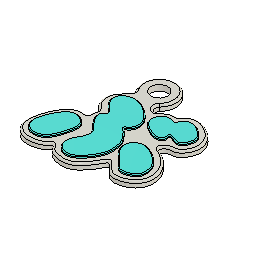
Azusa Keychain v20 (Autodesk Fusion 360 design; units mm, degrees)
Autodesk Fusion 360 part; units mm, degrees
sketch "bu body v1" plane through (0, 0, 0) normal (0, 0, 1) x (1, 0, 0)
  spline S0 degree 5 poles (6, 10.5) (6.0651, 10.4849) (6.1928, 10.4539) (6.3776, 10.4055) (6.613, 10.3384) (6.8974, 10.2472) (7.1797, 10.1429) (7.466, 10.0202) (7.7577, 9.8771) (8.05, 9.7182) (8.3341, 9.552) (8.6001, 9.3883) (8.8398, 9.2348) (9.05, 9.0947) (9.235, 8.9629) (9.4055, 8.8281) (9.573, 8.6777) (9.747, 8.5011) (9.9302, 8.2941) (10.1197, 8.0582) (10.3096, 7.798) (10.4927, 7.52) (10.6625, 7.2306) (10.8153, 6.9344) (10.9497, 6.6341) (11.0654, 6.3312) (11.1624, 6.0254) (11.2404, 5.7155) (11.2976, 5.3993) (11.3305, 5.0737) (11.3355, 4.7363) (11.3087, 4.3852) (11.2474, 4.0202) (11.1503, 3.6436) (11.0188, 3.2605) (10.8558, 2.8783) (10.6654, 2.5057) (10.4525, 2.1523) (10.2219, 1.8273) (9.9778, 1.5389) (9.7234, 1.2938) (9.4603, 1.0961) (9.1896, 0.9468) (8.9122, 0.8434) (8.6294, 0.7793) (8.3433, 0.743) (8.0573, 0.7185) (7.776, 0.6885) (7.5048, 0.638) (7.25, 0.557) (7.0183, 0.4446) (6.8165, 0.3081) (6.6486, 0.1589) (6.515, 0.0091) (6.4091, -0.1323) (6.3217, -0.2616) (6.2485, -0.3814) (6.1987, -0.5028) (6.1902, -0.6388) (6.2341, -0.7899) (6.3285, -0.9399) (6.4663, -1.0704) (6.6417, -1.1757) (6.8525, -1.2658) (7.0972, -1.3573) (7.3745, -1.4687) (7.6812, -1.612) (8.0118, -1.7924) (8.3596, -2.0101) (8.7171, -2.2614) (9.0767, -2.5407) (9.4313, -2.8418) (9.775, -3.1594) (10.1032, -3.4905) (10.413, -3.8338) (10.7021, -4.1895) (10.9689, -4.5584) (11.2124, -4.942) (11.4312, -5.3415) (11.624, -5.7579) (11.7883, -6.1909) (11.9216, -6.6394) (12.0205, -7.1012) (12.0818, -7.5733) (12.1022, -8.0519) (12.0791, -8.5327) (12.0101, -9.0107) (11.8939, -9.4807) (11.7303, -9.9369) (11.5201, -10.3736) (11.265, -10.7854) (10.9681, -11.1673) (10.6331, -11.5151) (10.265, -11.8256) (9.8696, -12.0971) (9.4537, -12.3293) (9.025, -12.5239) (8.5913, -12.6831) (8.1601, -12.8097) (7.7382, -12.9059) (7.331, -12.9733) (6.9418, -13.0114) (6.5716, -13.0176) (6.2187, -12.9866) (5.8795, -12.9125) (5.5505, -12.7901) (5.2287, -12.6178) (4.9132, -12.3982) (4.6064, -12.1412) (4.3142, -11.8637) (4.0441, -11.5857) (3.803, -11.3264) (3.595, -11.1004) (3.4204, -10.9147) (3.2725, -10.7632) (3.1384, -10.6297) (3.0052, -10.5012) (2.8642, -10.3791) (2.716, -10.2915) (2.5657, -10.2748) (2.4174, -10.3536) (2.2703, -10.5251) (2.1212, -10.7708) (1.9652, -11.0642) (1.7985, -11.3816) (1.6192, -11.7081) (1.427, -12.0355) (1.2221, -12.3604) (1.0058, -12.6828) (0.779, -13.0038) (0.5424, -13.3247) (0.2959, -13.6445) (0.0388, -13.9607) (-0.2302, -14.2697) (-0.5126, -14.5671) (-0.81, -14.848) (-1.1239, -15.1074) (-1.4556, -15.3407) (-1.8061, -15.5438) (-2.1756, -15.7134) (-2.5639, -15.8468) (-2.97, -15.9427) (-3.3917, -16.0007) (-3.8261, -16.0215) (-4.2689, -16.0076) (-4.7147, -15.9624) (-5.1574, -15.89) (-5.5901, -15.7943) (-6.0055, -15.6791) (-6.3959, -15.5471) (-6.7538, -15.3998) (-7.0715, -15.2363) (-7.3427, -15.0549) (-7.5644, -14.8549) (-7.7387, -14.638) (-7.8741, -14.41) (-7.9888, -14.1834) (-8.107, -13.9758) (-8.2489, -13.8056) (-8.4241, -13.6881) (-8.6195, -13.6311) (-8.8065, -13.6345) (-8.9599, -13.6934) (-9.078, -13.8005) (-9.1852, -13.9476) (-9.3132, -14.1249) (-9.485, -14.3213) (-9.7075, -14.5243) (-9.9776, -14.7218) (-10.2854, -14.9032) (-10.618, -15.0604) (-10.9635, -15.19) (-11.3136, -15.2929) (-11.6626, -15.3727) (-12.0072, -15.4345) (-12.3459, -15.4832) (-12.6791, -15.5221) (-13.008, -15.5512) (-13.3348, -15.5671) (-13.6619, -15.5645) (-13.9911, -15.5373) (-14.3239, -15.4801) (-14.6601, -15.389) (-14.9979, -15.2631) (-15.3341, -15.1035) (-15.6647, -14.9127) (-15.9847, -14.6934) (-16.2891, -14.4483) (-16.573, -14.179) (-16.8318, -13.8856) (-17.0613, -13.5667) (-17.2583, -13.2206) (-17.4199, -12.8452) (-17.544, -12.4388) (-17.6295, -12.0005) (-17.6761, -11.531) (-17.6844, -11.0324) (-17.6557, -10.508) (-17.5918, -9.9623) (-17.495, -9.4004) (-17.3677, -8.8281) (-17.2123, -8.2516) (-17.0313, -7.6772) (-16.8268, -7.1111) (-16.6005, -6.5593) (-16.3537, -6.0273) (-16.0876, -5.5203) (-15.8033, -5.0428) (-15.5022, -4.599) (-15.186, -4.1925) (-14.8569, -3.8264) (-14.5177, -3.503) (-14.1722, -3.2241) (-13.8251, -2.9907) (-13.4819, -2.8028) (-13.148, -2.6597) (-12.8282, -2.5589) (-12.5269, -2.4967) (-12.2466, -2.4675) (-11.9883, -2.4639) (-11.7515, -2.4769) (-11.5355, -2.4971) (-11.3399, -2.5147) (-11.1659, -2.5205) (-11.014, -2.508) (-10.8814, -2.4756) (-10.7587, -2.4294) (-10.6395, -2.3746) (-10.5367, -2.2995) (-10.4776, -2.1794) (-10.4711, -2.0027) (-10.4932, -1.7833) (-10.5096, -1.5453) (-10.4911, -1.3123) (-10.4352, -1.0926) (-10.3601, -0.8833) (-10.2924, -0.6772) (-10.2568, -0.4686) (-10.2659, -0.2603) (-10.3233, -0.0582) (-10.4256, 0.132) (-10.5661, 0.3095) (-10.7356, 0.4791) (-10.9244, 0.6487) (-11.1235, 0.8281) (-11.3257, 1.0264) (-11.5261, 1.2515) (-11.7209, 1.5098) (-11.9059, 1.8056) (-12.0764, 2.1406) (-12.2256, 2.5137) (-12.3447, 2.9206) (-12.4243, 3.3548) (-12.456, 3.8077) (-12.4336, 4.2692) (-12.3541, 4.7284) (-12.2194, 5.1739) (-12.0375, 5.5944) (-11.8227, 5.979) (-11.5921, 6.3193) (-11.3628, 6.6094) (-11.15, 6.8481) (-10.9635, 7.0391) (-10.8053, 7.1928) (-10.6677, 7.3267) (-10.5389, 7.4579) (-10.4069, 7.5986) (-10.2651, 7.7477) (-10.1137, 7.8962) (-9.9597, 8.0362) (-9.857, 8.18) (-9.8, 8.3) (-9.745, 8.49) (-9.7278, 8.731) (-9.7317, 8.9564) (-9.8441, 9.2185) (-9.9813, 9.4744) (-10.1241, 9.7107) (-10.2447, 9.9217) (-10.3356, 10.0776) (-10.3927, 10.1973) (-10.4249, 10.2758) (-10.4373, 10.3081) knots 0 0 0 0 0 0 0.00286533 0.00573066 0.00859599 0.01146132 0.01432665 0.01719198 0.02005731 0.02292264 0.02578797 0.0286533 0.03151862 0.03438395 0.03724928 0.04011461 0.04297994 0.04584527 0.0487106 0.05157593 0.05444126 0.05730659 0.06017192 0.06303725 0.06590258 0.06876791 0.07163324 0.07449857 0.0773639 0.08022923 0.08309456 0.08595989 0.08882521 0.09169054 0.09455587 0.0974212 0.10028653 0.10315186 0.10601719 0.10888252 0.11174785 0.11461318 0.11747851 0.12034384 0.12320917 0.1260745 0.12893983 0.13180516 0.13467049 0.13753582 0.14040115 0.14326648 0.14613181 0.14899713 0.15186246 0.15472779 0.15759312 0.16045845 0.16332378 0.16618911 0.16905444 0.17191977 0.1747851 0.17765043 0.18051576 0.18338109 0.18624642 0.18911175 0.19197708 0.19484241 0.19770774 0.20057307 0.2034384 0.20630372 0.20916905 0.21203438 0.21489971 0.21776504 0.22063037 0.2234957 0.22636103 0.22922636 0.23209169 0.23495702 0.23782235 0.24068768 0.24355301 0.24641834 0.24928367 0.252149 0.25501433 0.25787966 0.26074499 0.26361032 0.26647564 0.26934097 0.2722063 0.27507163 0.27793696 0.28080229 0.28366762 0.28653295 0.28939828 0.29226361 0.29512894 0.29799427 0.3008596 0.30372493 0.30659026 0.30945559 0.31232092 0.31518625 0.31805158 0.32091691 0.32378223 0.32664756 0.32951289 0.33237822 0.33524355 0.33810888 0.34097421 0.34383954 0.34670487 0.3495702 0.35243553 0.35530086 0.35816619 0.36103152 0.36389685 0.36676218 0.36962751 0.37249284 0.37535817 0.3782235 0.38108883 0.38395415 0.38681948 0.38968481 0.39255014 0.39541547 0.3982808 0.40114613 0.40401146 0.40687679 0.40974212 0.41260745 0.41547278 0.41833811 0.42120344 0.42406877 0.4269341 0.42979943 0.43266476 0.43553009 0.43839542 0.44126074 0.44412607 0.4469914 0.44985673 0.45272206 0.45558739 0.45845272 0.46131805 0.46418338 0.46704871 0.46991404 0.47277937 0.4756447 0.47851003 0.48137536 0.48424069 0.48710602 0.48997135 0.49283668 0.49570201 0.49856734 0.50143266 0.50429799 0.50716332 0.51002865 0.51289398 0.51575931 0.51862464 0.52148997 0.5243553 0.52722063 0.53008596 0.53295129 0.53581662 0.53868195 0.54154728 0.54441261 0.54727794 0.55014327 0.5530086 0.55587393 0.55873926 0.56160458 0.56446991 0.56733524 0.57020057 0.5730659 0.57593123 0.57879656 0.58166189 0.58452722 0.58739255 0.59025788 0.59312321 0.59598854 0.59885387 0.6017192 0.60458453 0.60744986 0.61031519 0.61318052 0.61604585 0.61891117 0.6217765 0.62464183 0.62750716 0.63037249 0.63323782 0.63610315 0.63896848 0.64183381 0.64469914 0.64756447 0.6504298 0.65329513 0.65616046 0.65902579 0.66189112 0.66475645 0.66762178 0.67048711 0.67335244 0.67621777 0.67908309 0.68194842 0.68481375 0.68767908 0.69054441 0.69340974 0.69627507 0.6991404 0.70200573 0.70487106 0.70773639 0.71060172 0.71346705 0.71633238 0.71919771 0.72206304 0.72492837 0.7277937 0.73065903 0.73352436 0.73638968 0.73925501 0.74212034 0.74498567 0.747851 0.75071633 0.75358166 0.75644699 0.75931232 0.76217765 0.76504298 0.76790831 0.77077364 0.77363897 0.7765043 0.77936963 0.78223496 0.78510029 0.78796562 0.79083095 0.79369628 0.79563186 0.79563186 0.79563186 0.79563186 0.79563186 0.79563186
  spline S1 degree 5 poles (-3.3703, 9.0276) (-3.381, 9.0158) (-3.4138, 8.9797) (-3.4691, 8.9165) (-3.5512, 8.8116) (-3.65, 8.65) (-3.6951, 8.4217) (-3.7207, 8.1798) (-3.6788, 7.9044) (-3.5655, 7.6182) (-3.3861, 7.3491) (-3.1557, 7.123) (-2.8982, 6.9575) (-2.6471, 6.8539) (-2.436, 6.8022) (-2.285, 6.7911) (-2.1899, 6.8154) (-2.1093, 6.8846) (-1.9979, 7.0086) (-1.8382, 7.1828) (-1.6328, 7.393) (-1.3945, 7.6201) (-1.1381, 7.8446) (-0.8694, 8.0524) (-0.5856, 8.2353) (-0.2811, 8.3893) (0.0484, 8.5132) (0.401, 8.6078) (0.7641, 8.6744) (1.1095, 8.7132) (1.4051, 8.7268) (1.626, 8.7231) (1.765, 8.7176) (1.8465, 8.7381) (1.9263, 8.8217) (2.0517, 8.9877) (2.2451, 9.2284) (2.5124, 9.5201) (2.8461, 9.8284) (3.2304, 10.1171) (3.6459, 10.3546) (4.0742, 10.5226) (4.5004, 10.6184) (4.9132, 10.6491) (5.3042, 10.6288) (5.5959, 10.5852) (5.8024, 10.5444) (5.9349, 10.5151) (6, 10.5) knots 0.875389 0.875389 0.875389 0.875389 0.875389 0.875389 0.876791 0.879656 0.882521 0.885387 0.888252 0.891117 0.893983 0.896848 0.899713 0.902579 0.905444 0.908309 0.911175 0.91404 0.916905 0.919771 0.922636 0.925501 0.928367 0.931232 0.934097 0.936963 0.939828 0.942693 0.945559 0.948424 0.951289 0.954155 0.95702 0.959885 0.962751 0.965616 0.968481 0.971347 0.974212 0.977077 0.979943 0.982808 0.985673 0.988539 0.991404 0.994269 0.997135 1 1 1 1 1 1
  arc A0 (-3.3703, 9.0276) -> (-10.2449, 9.9216) centre (-6.474, 12.0397) ccw
  circle A1 centre (-6.474, 12.0397) radius 2.1568
  point P0 (-10.4373, 10.3081)
  constraint coincident P0 A0
  constraint coincident S0 A0.end
  constraint concentric A0 A1
extrude "Extrude1" add sketch "bu body v1" along normal blind 1.5 contours S0 S1 A0
fillet "Fillet1" radius 0.5 3 edges at (-5.9163, 16.3285, 1.5) (-2.5581, -15.8345, 1.5) (-0.5045, 8.2701, 1.5)
sketch "bu middle v1" plane through (0, 0, 1.5) normal (0, 0, 1) x (1, 0, 0)
  spline S0 degree 5 poles (-1.4999, -2.0615) (-1.4521, -2.1021) (-1.322, -2.2306) (-1.044, -2.5481) (-0.6778, -2.9696) (-0.2817, -3.4492) (0.0829, -3.9373) (0.3768, -4.3995) (0.5894, -4.8223) (0.7286, -5.2064) (0.8143, -5.563) (0.8704, -5.9091) (0.9184, -6.2631) (0.9683, -6.6396) (1.017, -7.048) (1.0539, -7.4934) (1.0632, -7.9766) (1.0285, -8.4949) (0.9356, -9.0427) (0.7771, -9.6116) (0.5538, -10.1915) (0.2725, -10.7708) (-0.0555, -11.3373) (-0.4164, -11.879) (-0.7956, -12.3849) (-1.1794, -12.8453) (-1.5568, -13.2529) (-1.9215, -13.6035) (-2.273, -13.8964) (-2.6146, -14.1332) (-2.952, -14.3172) (-3.2914, -14.4522) (-3.6375, -14.5415) (-3.992, -14.587) (-4.3524, -14.5885) (-4.7141, -14.5456) (-5.0707, -14.4578) (-5.4157, -14.3258) (-5.7436, -14.1527) (-6.0503, -13.9438) (-6.3321, -13.7053) (-6.5857, -13.4427) (-6.8075, -13.1599) (-6.9927, -12.8578) (-7.1356, -12.5336) (-7.2314, -12.1851) (-7.2771, -11.8123) (-7.2732, -11.4202) (-7.2252, -11.0224) (-7.1435, -10.6398) (-7.04, -10.2937) (-6.9262, -9.9999) (-6.8104, -9.7632) (-6.6944, -9.5691) (-6.5746, -9.3869) (-6.4458, -9.1836) (-6.3055, -8.9353) (-6.1572, -8.6393) (-6.0094, -8.3067) (-5.8732, -7.9558) (-5.7618, -7.6061) (-5.6881, -7.2702) (-5.6638, -6.9502) (-5.6978, -6.6424) (-5.7949, -6.3396) (-5.9548, -6.0356) (-6.1697, -5.7279) (-6.4271, -5.4179) (-6.7114, -5.1081) (-7.007, -4.801) (-7.3, -4.4976) (-7.5813, -4.195) (-7.8475, -3.8862) (-8.0975, -3.5632) (-8.3304, -3.219) (-8.5425, -2.85) (-8.7254, -2.4587) (-8.8624, -2.0562) (-8.9319, -1.6607) (-8.9158, -1.2916) (-8.8068, -0.9655) (-8.6146, -0.6915) (-8.376, -0.4656) (-8.1494, -0.2713) (-7.996, -0.0868) (-7.9661, 0.111) (-8.08, 0.3395) (-8.3267, 0.6091) (-8.6751, 0.9243) (-9.0816, 1.2843) (-9.4994, 1.684) (-9.8869, 2.1143) (-10.2166, 2.5631) (-10.4728, 3.0167) (-10.6496, 3.4611) (-10.7483, 3.8836) (-10.7755, 4.274) (-10.7405, 4.6257) (-10.6533, 4.9382) (-10.5229, 5.2158) (-10.3572, 5.4651) (-10.162, 5.6936) (-9.9406, 5.9064) (-9.6933, 6.1054) (-9.4187, 6.2899) (-9.1145, 6.4564) (-8.7787, 6.5999) (-8.4102, 6.714) (-8.0096, 6.7914) (-7.5789, 6.8251) (-7.1209, 6.809) (-6.6398, 6.7387) (-6.1406, 6.6123) (-5.629, 6.4313) (-5.1118, 6.2001) (-4.5957, 5.9249) (-4.0883, 5.6133) (-3.5968, 5.2733) (-3.1288, 4.9124) (-2.6912, 4.5374) (-2.2908, 4.1529) (-1.9336, 3.7615) (-1.625, 3.3642) (-1.369, 2.9618) (-1.1685, 2.5555) (-1.0248, 2.1482) (-0.9375, 1.7447) (-0.9041, 1.3538) (-0.92, 0.986) (-0.9783, 0.6514) (-1.0696, 0.3562) (-1.1399, 0.1323) (-1.25, -0.1) (-1.322, -0.2268) (-1.45, -0.45) (-1.6, -0.6) (-1.7774, -0.7805) (-1.9546, -0.9373) (-2.216, -1.0792) (-2.3884, -1.1671) (-2.3804, -1.3192) (-2.1681, -1.5425) (-1.8622, -1.773) (-1.7, -1.9) (-1.5579, -2.0137) (-1.4999, -2.0615) knots 0 0 0 0 0 0 0.0070922 0.0141844 0.0212766 0.02836879 0.03546099 0.04255319 0.04964539 0.05673759 0.06382979 0.07092199 0.07801418 0.08510638 0.09219858 0.09929078 0.10638298 0.11347518 0.12056738 0.12765957 0.13475177 0.14184397 0.14893617 0.15602837 0.16312057 0.17021277 0.17730496 0.18439716 0.19148936 0.19858156 0.20567376 0.21276596 0.21985816 0.22695035 0.23404255 0.24113475 0.24822695 0.25531915 0.26241135 0.26950355 0.27659574 0.28368794 0.29078014 0.29787234 0.30496454 0.31205674 0.31914894 0.32624113 0.33333333 0.34042553 0.34751773 0.35460993 0.36170213 0.36879433 0.37588652 0.38297872 0.39007092 0.39716312 0.40425532 0.41134752 0.41843972 0.42553191 0.43262411 0.43971631 0.44680851 0.45390071 0.46099291 0.46808511 0.4751773 0.4822695 0.4893617 0.4964539 0.5035461 0.5106383 0.5177305 0.5248227 0.53191489 0.53900709 0.54609929 0.55319149 0.56028369 0.56737589 0.57446809 0.58156028 0.58865248 0.59574468 0.60283688 0.60992908 0.61702128 0.62411348 0.63120567 0.63829787 0.64539007 0.65248227 0.65957447 0.66666667 0.67375887 0.68085106 0.68794326 0.69503546 0.70212766 0.70921986 0.71631206 0.72340426 0.73049645 0.73758865 0.74468085 0.75177305 0.75886525 0.76595745 0.77304965 0.78014184 0.78723404 0.79432624 0.80141844 0.80851064 0.81560284 0.82269504 0.82978723 0.83687943 0.84397163 0.85106383 0.85815603 0.86524823 0.87234043 0.87943262 0.88652482 0.89361702 0.90070922 0.90780142 0.91489362 0.92198582 0.92907801 0.93617021 0.94326241 0.95035461 0.95744681 0.96453901 0.97163121 0.9787234 0.9858156 0.9929078 1 1 1 1 1 1
extrude "Extrude2" add sketch "bu middle v1" along normal blind 0.5
fillet "Fillet2" radius 0.22 1 edges at (-7.9705, -3.7225, 2)
sketch "bu left" plane through (0, 0, 1.5) normal (0, 0, 1) x (1, 0, 0)
  spline S0 degree 5 poles (-11.2319, -4.2705) (-11.3368, -4.247) (-11.5459, -4.2101) (-11.8552, -4.1859) (-12.2529, -4.2185) (-12.7189, -4.3651) (-13.1524, -4.6095) (-13.5556, -4.94) (-13.9323, -5.3437) (-14.2863, -5.8077) (-14.6209, -6.3198) (-14.9379, -6.8693) (-15.2367, -7.4474) (-15.5133, -8.0484) (-15.7606, -8.6685) (-15.969, -9.3042) (-16.1266, -9.9508) (-16.2204, -10.6009) (-16.2362, -11.2428) (-16.1596, -11.8595) (-15.979, -12.4317) (-15.6879, -12.9399) (-15.2872, -13.3667) (-14.7884, -13.6992) (-14.2146, -13.9304) (-13.595, -14.0572) (-12.9611, -14.079) (-12.3421, -13.9961) (-11.7608, -13.808) (-11.23, -13.5126) (-10.7555, -13.109) (-10.3375, -12.5995) (-9.9731, -11.9924) (-9.6573, -11.3039) (-9.3859, -10.5603) (-9.1556, -9.7939) (-8.9649, -9.0382) (-8.8153, -8.3236) (-8.7117, -7.6733) (-8.6634, -7.0985) (-8.6854, -6.5941) (-8.7937, -6.1445) (-9.0004, -5.7325) (-9.3099, -5.3458) (-9.7124, -4.9862) (-10.186, -4.6687) (-10.5995, -4.4653) (-10.9162, -4.3509) (-11.1269, -4.294) (-11.2319, -4.2705) knots 0 0 0 0 0 0 0.022222 0.044444 0.066667 0.088889 0.111111 0.133333 0.155556 0.177778 0.2 0.222222 0.244444 0.266667 0.288889 0.311111 0.333333 0.355556 0.377778 0.4 0.422222 0.444444 0.466667 0.488889 0.511111 0.533333 0.555556 0.577778 0.6 0.622222 0.644444 0.666667 0.688889 0.711111 0.733333 0.755556 0.777778 0.8 0.822222 0.844444 0.866667 0.888889 0.911111 0.933333 0.955556 0.977778 1 1 1 1 1 1
extrude "Extrude3" add sketch "bu left" along normal blind 0.5
fillet "Fillet3" radius 0.22 1 edges at (-13.9011, -13.9807, 2)
sketch "bu right v1" plane through (0, 0, 1.5) normal (0, 0, 1) x (1, 0, 0)
  spline S0 degree 5 poles (1.6702, -3.7585) (1.7162, -3.6884) (1.8146, -3.5514) (1.9804, -3.3553) (2.2323, -3.1151) (2.5811, -2.8566) (2.9472, -2.6459) (3.3181, -2.4885) (3.69, -2.3889) (4.0694, -2.3502) (4.4674, -2.3739) (4.8957, -2.4596) (5.3623, -2.605) (5.866, -2.8059) (6.398, -3.0561) (6.9441, -3.3483) (7.4873, -3.6746) (8.0096, -4.027) (8.4947, -4.398) (8.9304, -4.7812) (9.3094, -5.1715) (9.6285, -5.5652) (9.8882, -5.9598) (10.0922, -6.3547) (10.2466, -6.7503) (10.3597, -7.1489) (10.4393, -7.5533) (10.4901, -7.9656) (10.5109, -8.3862) (10.4916, -8.8126) (10.412, -9.2383) (10.2494, -9.6543) (9.9847, -10.0497) (9.6093, -10.413) (9.1325, -10.7324) (8.5844, -10.9976) (8.0057, -11.1994) (7.4411, -11.3309) (6.9308, -11.3879) (6.546, -11.3684) (6.2289, -11.2852) (5.9439, -11.1314) (5.7299, -10.938) (5.5217, -10.6792) (5.3, -10.4) (5.0277, -10.0638) (4.7561, -9.7529) (4.4497, -9.4429) (4.1122, -9.1368) (3.7514, -8.8313) (3.3779, -8.5198) (3.0042, -8.1943) (2.6432, -7.8473) (2.307, -7.4742) (2.0057, -7.0753) (1.7478, -6.6552) (1.5404, -6.221) (1.3895, -5.7812) (1.3007, -5.3445) (1.2795, -4.9179) (1.3305, -4.5069) (1.4308, -4.1946) (1.5387, -3.9716) (1.6243, -3.8285) (1.6702, -3.7585) knots 0 0 0 0 0 0 0.01666667 0.03333333 0.05 0.06666667 0.08333333 0.1 0.11666667 0.13333333 0.15 0.16666667 0.18333333 0.2 0.21666667 0.23333333 0.25 0.26666667 0.28333333 0.3 0.31666667 0.33333333 0.35 0.36666667 0.38333333 0.4 0.41666667 0.43333333 0.45 0.46666667 0.48333333 0.5 0.51666667 0.53333333 0.55 0.56666667 0.58333333 0.6 0.61666667 0.63333333 0.65 0.66666667 0.68333333 0.7 0.71666667 0.73333333 0.75 0.76666667 0.78333333 0.8 0.81666667 0.83333333 0.85 0.86666667 0.88333333 0.9 0.91666667 0.93333333 0.95 0.96666667 0.98333333 1 1 1 1 1 1
extrude "Extrude5" add sketch "bu right v1" along normal blind 0.5
fillet "Fillet5" radius 0.22 1 edges at (9.9572, -10.0417, 2)
sketch "bu top v1" plane through (0, 0, 1.5) normal (0, 0, 1) x (1, 0, 0)
  spline S0 degree 5 poles (-0.3764, 2.8228) (-0.3284, 2.7694) (-0.2283, 2.6637) (-0.0655, 2.5087) (0.1744, 2.3087) (0.5054, 2.0703) (0.8593, 1.8445) (1.2276, 1.6332) (1.602, 1.4387) (1.9753, 1.2641) (2.3418, 1.1127) (2.698, 0.9879) (3.0414, 0.8931) (3.3709, 0.8314) (3.6856, 0.8051) (3.9848, 0.8154) (4.2675, 0.8624) (4.5317, 0.9449) (4.7738, 1.0615) (4.9878, 1.2102) (5.1648, 1.39) (5.2921, 1.6006) (5.359, 1.8399) (5.3632, 2.1016) (5.3157, 2.3719) (5.249, 2.6269) (5.207, 2.8375) (5.232, 2.9779) (5.3522, 3.033) (5.5698, 3.0052) (5.8687, 2.9103) (6.2222, 2.772) (6.6008, 2.6181) (6.9804, 2.4748) (7.3455, 2.3643) (7.6862, 2.3039) (7.9977, 2.3053) (8.2783, 2.373) (8.5283, 2.5037) (8.7478, 2.6848) (8.9377, 2.8985) (9.0995, 3.1264) (9.2352, 3.3538) (9.3486, 3.5744) (9.4443, 3.7937) (9.5265, 4.0221) (9.5977, 4.2714) (9.6572, 4.549) (9.6994, 4.853) (9.7158, 5.1751) (9.6972, 5.503) (9.6356, 5.824) (9.5264, 6.1277) (9.3707, 6.4094) (9.1742, 6.6696) (8.9452, 6.9121) (8.6921, 7.1426) (8.4221, 7.3669) (8.1384, 7.5893) (7.8394, 7.8117) (7.5212, 8.033) (7.179, 8.2498) (6.8086, 8.4433) (6.4, 8.6) (6, 8.7) (5.4962, 8.7762) (5.1, 8.75) (4.8, 8.7) (4.5, 8.6) (4.15, 8.4) (3.9, 8.2) (3.7, 8) (3.45, 7.69) (3.3, 7.45) (3.1259, 7.1354) (2.9739, 6.5794) (3.2319, 6.5876) (2.75, 6.75) (2.5, 6.85) (2.3, 6.9) (2.1, 6.95) (1.8232, 6.9836) (1.6, 7) (1.3377, 7.0095) (1.1309, 7.0073) (0.923, 6.9828) (0.7101, 6.9367) (0.49, 6.8687) (0.2642, 6.775) (0.0377, 6.6487) (-0.1827, 6.4828) (-0.3889, 6.272) (-0.5738, 6.0153) (-0.7313, 5.7179) (-0.857, 5.3894) (-0.9473, 5.042) (-0.9992, 4.6883) (-1.0104, 4.3394) (-0.9785, 4.0031) (-0.9013, 3.6831) (-0.7771, 3.3801) (-0.6397, 3.1505) (-0.5158, 2.9844) (-0.4243, 2.8763) (-0.3764, 2.8228) knots 0 0 0 0 0 0 0.01 0.02 0.03 0.04 0.05 0.06 0.07 0.08 0.09 0.1 0.11 0.12 0.13 0.14 0.15 0.16 0.17 0.18 0.19 0.2 0.21 0.22 0.23 0.24 0.25 0.26 0.27 0.28 0.29 0.3 0.31 0.32 0.33 0.34 0.35 0.36 0.37 0.38 0.39 0.4 0.41 0.42 0.43 0.44 0.45 0.46 0.47 0.48 0.49 0.5 0.51 0.52 0.53 0.54 0.55 0.56 0.57 0.58 0.59 0.6 0.61 0.62 0.63 0.64 0.65 0.66 0.67 0.68 0.69 0.7 0.71 0.72 0.73 0.74 0.75 0.76 0.77 0.78 0.79 0.8 0.81 0.82 0.83 0.84 0.85 0.86 0.87 0.88 0.89 0.9 0.91 0.92 0.93 0.94 0.95 0.96 0.97 0.98 0.99 1 1 1 1 1 1
extrude "Extrude6" add sketch "bu top v1" along normal blind 0.5
fillet "Fillet6" radius 0.22 1 edges at (9.5148, 6.1222, 2)
